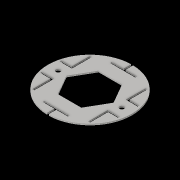
# Autodesk Inventor part: Luxcan centrador lente 38
Saved by Autodesk Inventor 2016 (Build 200138000, 138)
## iProperties
Created: 2018-08-10
Part Number: Luxcan centrador lente 38
Material: Generic
Document SubType Name: Sheet Metal
Designer: jocdurso
Density: 1 g/cm^3
Sheet Metal Rule: Default
Appearance: Default
Author: jocdurso
Autodesk Inventor part; units mm, degrees
ref_plane "YZ Plane" through (0, 0, 0) normal (1, 0, 0) x (0, 1, 0)
ref_plane "XZ Plane" through (0, 0, 0) normal (0, 1, 0) x (-1, 0, 0)
ref_plane "XY Plane" through (0, 0, 0) normal (0, 0, 1) x (1, 0, 0)
sketch "Sketch1" plane through (0, 0, 0) normal (0, 1, 0) x (-1, 0, 0)
  circle A0 centre (0, 0) radius 29
  line L0 (-8.1695, -14.15) -> (-16.339, 0)
  line L1 (-16.339, 0) -> (-8.1695, 14.15)
  line L2 (-8.1695, 14.15) -> (8.1695, 14.15)
  line L3 (8.1695, 14.15) -> (16.339, 0)
  line L4 (16.339, 0) -> (8.1695, -14.15)
  line L5 (8.1695, -14.15) -> (-8.1695, -14.15)
  dimension "d0" = 58
  dimension "d1" = 28.3
  measures "d0" diameter of A0
  measures "d1" distance between parallel lines of L2 L5
extrude "Plate1" add sketch "Sketch1" along normal blind 1
sketch "Sketch2" plane through (0, 0, 0) normal (0, 1, 0) x (-1, 0, 0)
  point P0 (0, 0)
  point P1 (22, 0)
  point P2 (-22, 0)
  dimension "d3" = 22
  dimension "d4" = 22
  constraints: 2 horizontal alignment
  measures "d3" distance of point (0, 0) point (22, 0)
  measures "d4" distance of point (-22, 0) point (0, 0)
hole "Hole1" at (-22, 0, 0) at (22, 0, 0) direction (0, 1, 0) diameter 3.3 end through all
sketch "Sketch3" plane through (0, 1, 0) normal (0, 1, 0) x (1, 0, 0)
  line L0 (0, 0) -> (8.5176, 0)
  line L1 (0, 0) -> (0, 7.5276)
  line L2 (-8.75, 24) -> (8.75, 24)
  line L3 (8.75, 24) -> (8.75, 22.5)
  line L4 (8.75, 22.5) -> (-8.75, 22.5)
  line L5 (-8.75, 22.5) -> (-8.75, 24)
  line L6 (0.75, 42.5) -> (-0.75, 42.5)
  line L7 (-0.75, 42.5) -> (-0.75, 22.5)
  line L8 (-0.75, 22.5) -> (0.75, 22.5)
  line L9 (0.75, 22.5) -> (0.75, 42.5)
  line L10 (-8.75, -24) -> (8.75, -24)
  line L11 (8.75, -24) -> (8.75, -22.5)
  line L12 (8.75, -22.5) -> (-8.75, -22.5)
  line L13 (-8.75, -22.5) -> (-8.75, -24)
  line L14 (0.75, -42.5) -> (-0.75, -42.5)
  line L15 (-0.75, -42.5) -> (-0.75, -22.5)
  line L16 (-0.75, -22.5) -> (0.75, -22.5)
  line L17 (0.75, -22.5) -> (0.75, -42.5)
  line L18 (-27, 7.5) -> (-18.5, 7.5)
  line L19 (-18.5, 7.5) -> (-18.5, 6)
  line L20 (-18.5, 6) -> (-27, 6)
  line L21 (-27, 6) -> (-27, 7.5)
  line L22 (-18.5, 6) -> (-20, 6)
  line L23 (-20, 6) -> (-20, 20)
  line L24 (-20, 20) -> (-18.5, 20)
  line L25 (-18.5, 20) -> (-18.5, 6)
  line L26 (27, 7.5) -> (18.5, 7.5)
  line L27 (18.5, 7.5) -> (18.5, 6)
  line L28 (18.5, 6) -> (27, 6)
  line L29 (27, 6) -> (27, 7.5)
  line L30 (18.5, 6) -> (20, 6)
  line L31 (20, 6) -> (20, 20)
  line L32 (20, 20) -> (18.5, 20)
  line L33 (18.5, 20) -> (18.5, 6)
  line L34 (-27, -7.5) -> (-18.5, -7.5)
  line L35 (-18.5, -7.5) -> (-18.5, -6)
  line L36 (-18.5, -6) -> (-27, -6)
  line L37 (-27, -6) -> (-27, -7.5)
  line L38 (-18.5, -6) -> (-20, -6)
  line L39 (-20, -6) -> (-20, -20)
  line L40 (-20, -20) -> (-18.5, -20)
  line L41 (-18.5, -20) -> (-18.5, -6)
  line L42 (18.5, -20) -> (18.5, -6)
  line L43 (20, -6) -> (20, -20)
  line L44 (20, -20) -> (18.5, -20)
  line L45 (18.5, -7.5) -> (18.5, -6)
  line L46 (18.5, -6) -> (20, -6)
  line L47 (27, -6) -> (27, -7.5)
  line L48 (27, -7.5) -> (18.5, -7.5)
  line L49 (18.5, -6) -> (27, -6)
  point P0 (0, 22.5)
  point P1 (0, -22.5)
  dimension "d12" = 1.5
  dimension "d13" = 1.5
  dimension "d14" = 22.5
  dimension "d15" = 17.5
  dimension "d16" = 20
  dimension "d17" = 1.5
  dimension "d18" = 1.5
  dimension "d19" = 8.5
  dimension "d20" = 14
  dimension "d21" = 6
  dimension "d22" = 18.5
  constraints: 100 end point, 30 symmetric about line, 8 parallel, 5 horizontal, 4 perpendicular, 2 midpoint, 1 vertical, 1 vertical alignment
  measures "d12" distance of L6.start L6.end
  measures "d13" distance of L2.end L3.end
  measures "d14" distance between parallel lines of L0 L4
  measures "d15" distance of L3.end L4.end
  measures "d16" distance of L8.end L6.start
  measures "d17" distance of L20.end L18.start
  measures "d18" distance of L23.end L24.end
  measures "d19" distance between parallel lines of L25 L21
  measures "d20" distance between parallel lines of L24 L20
  measures "d21" distance from line of L0.start L20
  measures "d22" distance from line of point (0, 22.5) L25
extrude "Cut1" cut sketch "Sketch3" against normal blind 1
equation "\"d10\" = Thickness"
equation "\"d23\" = Thickness"
equation "\"BendRadius\" = Thickness"
equation "\"BendReliefWidth\" = Thickness"
equation "\"BendReliefDepth\" = 0.5 * Thickness"
equation "\"CornerReliefSize\" = 4 * Thickness"
equation "\"MinimumRemnant\" = 2 * Thickness"
equation "\"TransitionRadius\" = BendRadius"
equation "\"JacobiRadiusSize\" = BendRadius"
equation "\"GapSize\" = Thickness"
equation "\"d2\" = BendRadius"
equation "\"Thickness\" = 1"
body "Solid1"
